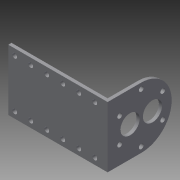
# Autodesk Inventor part: 知能ロボコンタミヤギヤードモータ用マウント
Saved by Autodesk Inventor 2013 (Build 170138000, 138)
## iProperties
Created: 2014-08-06
Part Number: 知能ロボコンタミヤギヤードモータ用マウント
Material: 一般
Document SubType Name: Modeling
Designer: horumo136
Density: 1 g/cm^3
Author: horumo136
Autodesk Inventor part; units mm, degrees
ref_plane "YZ Plane" through (0, 0, 0) normal (1, 0, 0) x (0, 1, 0)
ref_plane "XZ Plane" through (0, 0, 0) normal (0, 1, 0) x (-1, 0, 0)
ref_plane "XY Plane" through (0, 0, 0) normal (0, 0, 1) x (1, 0, 0)
sketch "スケッチ1" plane through (0, 0, 0) normal (0, 1, 0) x (-1, 0, 0)
  line L0 (0, 0) -> (-62, 0)
  line L1 (-62, 0) -> (-62, 38)
  line L2 (-62, 38) -> (0, 38)
  line L3 (0, 38) -> (0, 0)
  dimension "d0" = 62
  dimension "d1" = 38
  constraints: 8 end point, 2 parallel, 1 horizontal, 1 perpendicular
  measures "d0" distance of L1.end L2.end
  measures "d1" distance of L0.end L1.end
extrude "押し出し1" add sketch "スケッチ1" along normal blind 2
sketch "スケッチ2" plane through (0, 2, 0) normal (0, 1, 0) x (1, 0, 0)
  line L0 (0, 0) -> (0, -38) projected
  line L1 (62, -38) -> (62, 0) projected
  line L2 (0, 0) -> (4, 0)
  line L3 (4, 0) -> (4, -4)
  line L4 (4, -4) -> (0, -4)
  line L5 (0, -4) -> (0, 0)
  line L6 (4, -4) -> (14, -4)
  line L7 (14, -4) -> (24, -4)
  line L8 (24, -4) -> (34, -4)
  line L9 (34, -4) -> (44, -4)
  line L10 (44, -4) -> (54, -4)
  line L11 (0, -19) -> (62, -19)
  point P0 (4, -34)
  point P1 (14, -34)
  point P2 (24, -34)
  point P3 (34, -34)
  point P4 (44, -34)
  point P5 (54, -34)
  point P6 (4, -34)
  point P7 (14, -34)
  dimension "d4" = 4
  dimension "d5" = 4
  dimension "d6" = 10
  dimension "d7" = 10
  dimension "d8" = 10
  dimension "d9" = 10
  dimension "d10" = 10
  constraints: 20 end point, 10 coincident, 6 equal length, 6 symmetric about line, 2 midpoint, 2 perpendicular, 1 horizontal
  measures "d4" distance of L3.end L4.end
  measures "d5" distance of L2.end L3.end
  measures "d6" distance of L6.start L6.end
  measures "d7" distance of L6.end L7.end
  measures "d8" distance of L7.end L8.end
  measures "d9" distance of L8.end L9.end
  measures "d10" distance of L9.end L10.end
hole "穴1" at (4, 2, 4) at (14, 2, 4) at (24, 2, 4) at (34, 2, 4) at (44, 2, 4) at (54, 2, 4) at (24, 2, 34) at (34, 2, 34) at (44, 2, 34) at (54, 2, 34) at (4, 2, 34) at (14, 2, 34) direction (0, -1, 0) diameter 3 depth 8 tip angle 118
sketch "スケッチ3" plane through (0, 2, 0) normal (0, 1, 0) x (1, 0, 0)
  line L0 (0, -38) -> (62, -38) projected
  line L1 (62, -38) -> (62, 0) projected
  line L2 (62, 0) -> (60, 0)
  line L3 (60, 0) -> (60, -38)
  line L4 (60, -38) -> (62, -38)
  line L5 (62, -38) -> (62, 0)
  dimension "d18" = 2
  constraints: 8 end point, 2 parallel, 1 horizontal, 1 perpendicular, 1 point on line
  measures "d18" distance of L4.end L3.end
extrude "押し出し2" add sketch "スケッチ3" along normal blind 38
fillet "フィレット1" radius 19 2 edges at (61, 40, 38) (61, 40, 0)
sketch "スケッチ4" plane through (62, 0, 38) normal (1, 0, 0) x (0, 0, -1)
  arc A0 (38, 21) -> (0, 21) centre (19, 21) ccw projected
  line L0 (38, 0) -> (38, 21) projected
  circle A1 centre (19, 21) radius 15.5
  circle A2 centre (34.5, 21) radius 1.5
  circle A3 centre (26.75, 34.4234) radius 1.5
  circle A4 centre (11.25, 34.4234) radius 1.5
  circle A5 centre (3.5, 21) radius 1.5
  circle A6 centre (11.25, 7.5766) radius 1.5
  circle A7 centre (26.75, 7.5766) radius 1.5
  line L1 (19, 21) -> (19, 28)
  circle A8 centre (19, 28) radius 6
  line L2 (19, 21) -> (19, 14)
  circle A9 centre (19, 14) radius 6
  dimension "d22" = 31
  dimension "d23" = 3
  dimension "d26" = 360
  dimension "d28" = 7
  dimension "d29" = 12
  dimension "d30" = 7
  dimension "d31" = 12
  constraints: 8 centre point, 4 end point, 3 coincident, 1 collinear, 1 horizontal alignment, 1 parallel, 15 other
  measures "d23" diameter of A2
  measures "d28" distance of L1.start L1.end
  measures "d29" diameter of A8
  measures "d30" distance of L1.start L2.end
  measures "d31" diameter of A9
extrude "押し出し3" cut sketch "スケッチ4" against normal blind 3 contours A1 A2 | A1 A2 | A3 A1 | A1 A3 | A7 A1 | A1 A7 | A4 A1 | A1 A4 | A6 A1 | A1 A6 | A5 A1 | A1 A5 | A8 | A9
